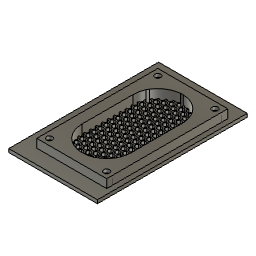
cover_side v6 (Autodesk Fusion 360 design; units mm, degrees)
Autodesk Fusion 360 part; units mm, degrees
(part 1 of 2)
sketch "Skizze1" plane through (0, 0, 0) normal (0, 0, 1) x (1, 0, 0)
  line L0 (26, -43.9) -> (-26, 43.9) construction
  line L1 (-26, -43.9) -> (26, 43.9) construction
  line L2 (21, -35.5) -> (-21, 35.5) construction
  line L3 (-21, -35.5) -> (21, 35.5) construction
  line L4 (23, -37.5) -> (-23, 37.5) construction
  line L5 (-23, -37.5) -> (23, 37.5) construction
  line L6 (0, 60) -> (0, -55) construction
  line L7 (16.75, -31.75) -> (-16.75, -31.75) construction
  line L8 (-16.75, -31.75) -> (-16.75, 31.75) construction
  line L9 (-16.75, 31.75) -> (16.75, 31.75) construction
  line L10 (16.75, 31.75) -> (16.75, -31.75) construction
  line L11 (16.75, -31.75) -> (-16.75, 31.75) construction
  line L12 (-16.75, -31.75) -> (16.75, 31.75) construction
  line L13 (20.5, -35.5) -> (-20.5, -35.5)
  line L14 (-20.5, -35.5) -> (-20.5, 35.5)
  line L15 (-20.5, 35.5) -> (20.5, 35.5)
  line L16 (20.5, 35.5) -> (20.5, -35.5)
  line L17 (20.5, -35.5) -> (-20.5, 35.5) construction
  line L18 (-20.5, -35.5) -> (20.5, 35.5) construction
  line L19 (-34.4017, -15) -> (37.5784, -15) construction
  line L20 (-32.2154, 15) -> (36.7375, 15) construction
  line L21 (14.5, -29.5) -> (-14.5, -29.5) construction
  line L22 (-14.5, -29.5) -> (-14.5, 29.5) construction
  line L23 (-14.5, 29.5) -> (14.5, 29.5) construction
  line L24 (14.5, 29.5) -> (14.5, -29.5) construction
  line L25 (14.5, -29.5) -> (-14.5, 29.5) construction
  line L26 (-14.5, -29.5) -> (14.5, 29.5) construction
  arc A0 (14.5, 15) -> (-14.5, 15) centre (0, 15) ccw
  arc A1 (-14.5, -15) -> (14.5, -15) centre (0, -15) ccw
  line L27 (-14.5, -15) -> (-14.5, 15)
  line L28 (14.5, -15) -> (14.5, 15)
  line L29 (-13.75, -30.799) -> (-13, -29.5)
  line L30 (-13, -29.5) -> (-13.75, -28.201)
  line L31 (-13.75, -28.201) -> (-15.25, -28.201)
  line L32 (-15.25, -28.201) -> (-16, -29.5)
  line L33 (-16, -29.5) -> (-15.25, -30.799)
  line L34 (-15.25, -30.799) -> (-13.75, -30.799)
  line L35 (-11.673, -26.8) -> (-11.673, -30.7) construction
  line L36 (-15, -27.75) -> (-9.3, -27.75) construction
  line L37 (-10.923, -29.049) -> (-10.173, -27.75)
  line L38 (-10.173, -27.75) -> (-10.923, -26.451)
  line L39 (-10.923, -26.451) -> (-12.423, -26.451)
  line L40 (-12.423, -26.451) -> (-13.173, -27.75)
  line L41 (-13.173, -27.75) -> (-12.423, -29.049)
  line L42 (-12.423, -29.049) -> (-10.923, -29.049)
  line L43 (-7.3455, -29.5) -> (-8.0955, -28.201)
  line L44 (-8.0955, -28.201) -> (-9.5955, -28.201)
  line L45 (-9.5955, -28.201) -> (-10.3455, -29.5)
  line L46 (-10.3455, -29.5) -> (-9.5955, -30.799)
  line L47 (-9.5955, -30.799) -> (-8.0955, -30.799)
  line L48 (-8.0955, -30.799) -> (-7.3455, -29.5)
  line L49 (-4.5185, -27.75) -> (-5.2685, -26.451)
  line L50 (-5.2685, -26.451) -> (-6.7685, -26.451)
  line L51 (-6.7685, -26.451) -> (-7.5185, -27.75)
  line L52 (-7.5185, -27.75) -> (-6.7685, -29.049)
  line L53 (-5.2685, -29.049) -> (-4.5185, -27.75)
  line L54 (-6.7685, -29.049) -> (-5.2685, -29.049)
  line L55 (-1.691, -29.5) -> (-2.441, -28.201)
  line L56 (-2.441, -28.201) -> (-3.941, -28.201)
  line L57 (-3.941, -28.201) -> (-4.691, -29.5)
  line L58 (-4.691, -29.5) -> (-3.941, -30.799)
  line L59 (-3.941, -30.799) -> (-2.441, -30.799)
  line L60 (-2.441, -30.799) -> (-1.691, -29.5)
  line L61 (1.136, -27.75) -> (0.386, -26.451)
  line L62 (0.386, -26.451) -> (-1.114, -26.451)
  line L63 (-1.114, -26.451) -> (-1.864, -27.75)
  line L64 (-1.864, -27.75) -> (-1.114, -29.049)
  line L65 (0.386, -29.049) -> (1.136, -27.75)
  line L66 (-1.114, -29.049) -> (0.386, -29.049)
  line L67 (3.9635, -29.5) -> (3.2135, -28.201)
  line L68 (3.2135, -28.201) -> (1.7135, -28.201)
  line L69 (1.7135, -28.201) -> (0.9635, -29.5)
  line L70 (0.9635, -29.5) -> (1.7135, -30.799)
  line L71 (1.7135, -30.799) -> (3.2135, -30.799)
  line L72 (3.2135, -30.799) -> (3.9635, -29.5)
  line L73 (6.7905, -27.75) -> (6.0405, -26.451)
  line L74 (6.0405, -26.451) -> (4.5405, -26.451)
  line L75 (4.5405, -26.451) -> (3.7905, -27.75)
  line L76 (3.7905, -27.75) -> (4.5405, -29.049)
  line L77 (6.0405, -29.049) -> (6.7905, -27.75)
  line L78 (4.5405, -29.049) -> (6.0405, -29.049)
  line L79 (9.618, -29.5) -> (8.868, -28.201)
  line L80 (8.868, -28.201) -> (7.368, -28.201)
  line L81 (7.368, -28.201) -> (6.618, -29.5)
  line L82 (6.618, -29.5) -> (7.368, -30.799)
  line L83 (7.368, -30.799) -> (8.868, -30.799)
  line L84 (8.868, -30.799) -> (9.618, -29.5)
  line L85 (12.445, -27.75) -> (11.695, -26.451)
  line L86 (11.695, -26.451) -> (10.195, -26.451)
  line L87 (10.195, -26.451) -> (9.445, -27.75)
  line L88 (9.445, -27.75) -> (10.195, -29.049)
  line L89 (11.695, -29.049) -> (12.445, -27.75)
  line L90 (10.195, -29.049) -> (11.695, -29.049)
  line L91 (15.2725, -29.5) -> (14.5225, -28.201)
  line L92 (14.5225, -28.201) -> (13.0225, -28.201)
  line L93 (13.0225, -28.201) -> (12.2725, -29.5)
  line L94 (12.2725, -29.5) -> (13.0225, -30.799)
  line L95 (13.0225, -30.799) -> (14.5225, -30.799)
  line L96 (14.5225, -30.799) -> (15.2725, -29.5)
  line L97 (18.0995, -27.75) -> (17.3495, -26.451)
  line L98 (17.3495, -26.451) -> (15.8495, -26.451)
  line L99 (15.8495, -26.451) -> (15.0995, -27.75)
  line L100 (15.0995, -27.75) -> (15.8495, -29.049)
  line L101 (17.3495, -29.049) -> (18.0995, -27.75)
  line L102 (15.8495, -29.049) -> (17.3495, -29.049)
  line L103 (-13, -26) -> (-13.75, -24.701)
  line L104 (-13.75, -24.701) -> (-15.25, -24.701)
  line L105 (-15.25, -24.701) -> (-16, -26)
  line L106 (-16, -26) -> (-15.25, -27.299)
  line L107 (-15.25, -27.299) -> (-13.75, -27.299)
  line L108 (-13.75, -27.299) -> (-13, -26)
  line L109 (-10.173, -24.25) -> (-10.923, -22.951)
  line L110 (-10.923, -22.951) -> (-12.423, -22.951)
  line L111 (-12.423, -22.951) -> (-13.173, -24.25)
  line L112 (-13.173, -24.25) -> (-12.423, -25.549)
  line L113 (-10.923, -25.549) -> (-10.173, -24.25)
  line L114 (-12.423, -25.549) -> (-10.923, -25.549)
  line L115 (-7.3455, -26) -> (-8.0955, -24.701)
  line L116 (-8.0955, -24.701) -> (-9.5955, -24.701)
  line L117 (-9.5955, -24.701) -> (-10.3455, -26)
  line L118 (-10.3455, -26) -> (-9.5955, -27.299)
  line L119 (-9.5955, -27.299) -> (-8.0955, -27.299)
  line L120 (-8.0955, -27.299) -> (-7.3455, -26)
  line L121 (-4.5185, -24.25) -> (-5.2685, -22.951)
  line L122 (-5.2685, -22.951) -> (-6.7685, -22.951)
  line L123 (-6.7685, -22.951) -> (-7.5185, -24.25)
  line L124 (-7.5185, -24.25) -> (-6.7685, -25.549)
  line L125 (-5.2685, -25.549) -> (-4.5185, -24.25)
  line L126 (-6.7685, -25.549) -> (-5.2685, -25.549)
  line L127 (-1.691, -26) -> (-2.441, -24.701)
  line L128 (-2.441, -24.701) -> (-3.941, -24.701)
  line L129 (-3.941, -24.701) -> (-4.691, -26)
  line L130 (-4.691, -26) -> (-3.941, -27.299)
  line L131 (-3.941, -27.299) -> (-2.441, -27.299)
  line L132 (-2.441, -27.299) -> (-1.691, -26)
  line L133 (1.136, -24.25) -> (0.386, -22.951)
  line L134 (0.386, -22.951) -> (-1.114, -22.951)
  line L135 (-1.114, -22.951) -> (-1.864, -24.25)
  line L136 (-1.864, -24.25) -> (-1.114, -25.549)
  line L137 (0.386, -25.549) -> (1.136, -24.25)
  line L138 (-1.114, -25.549) -> (0.386, -25.549)
  line L139 (3.9635, -26) -> (3.2135, -24.701)
  line L140 (3.2135, -24.701) -> (1.7135, -24.701)
  line L141 (1.7135, -24.701) -> (0.9635, -26)
  line L142 (0.9635, -26) -> (1.7135, -27.299)
  line L143 (1.7135, -27.299) -> (3.2135, -27.299)
  line L144 (3.2135, -27.299) -> (3.9635, -26)
  line L145 (6.7905, -24.25) -> (6.0405, -22.951)
  line L146 (6.0405, -22.951) -> (4.5405, -22.951)
  line L147 (4.5405, -22.951) -> (3.7905, -24.25)
  line L148 (3.7905, -24.25) -> (4.5405, -25.549)
  line L149 (6.0405, -25.549) -> (6.7905, -24.25)
  line L150 (4.5405, -25.549) -> (6.0405, -25.549)
  line L151 (9.618, -26) -> (8.868, -24.701)
  line L152 (8.868, -24.701) -> (7.368, -24.701)
  line L153 (7.368, -24.701) -> (6.618, -26)
  line L154 (6.618, -26) -> (7.368, -27.299)
  line L155 (7.368, -27.299) -> (8.868, -27.299)
  line L156 (8.868, -27.299) -> (9.618, -26)
  line L157 (12.445, -24.25) -> (11.695, -22.951)
  line L158 (11.695, -22.951) -> (10.195, -22.951)
  line L159 (10.195, -22.951) -> (9.445, -24.25)
  line L160 (9.445, -24.25) -> (10.195, -25.549)
  line L161 (11.695, -25.549) -> (12.445, -24.25)
  line L162 (10.195, -25.549) -> (11.695, -25.549)
  line L163 (15.2725, -26) -> (14.5225, -24.701)
  line L164 (14.5225, -24.701) -> (13.0225, -24.701)
  line L165 (13.0225, -24.701) -> (12.2725, -26)
  line L166 (12.2725, -26) -> (13.0225, -27.299)
  line L167 (13.0225, -27.299) -> (14.5225, -27.299)
  line L168 (14.5225, -27.299) -> (15.2725, -26)
  line L169 (18.0995, -24.25) -> (17.3495, -22.951)
  line L170 (17.3495, -22.951) -> (15.8495, -22.951)
  line L171 (15.8495, -22.951) -> (15.0995, -24.25)
  line L172 (15.0995, -24.25) -> (15.8495, -25.549)
  line L173 (17.3495, -25.549) -> (18.0995, -24.25)
  line L174 (15.8495, -25.549) -> (17.3495, -25.549)
  line L175 (-13, -22.5) -> (-13.75, -21.201)
  line L176 (-13.75, -21.201) -> (-15.25, -21.201)
  line L177 (-15.25, -21.201) -> (-16, -22.5)
  line L178 (-16, -22.5) -> (-15.25, -23.799)
  line L179 (-15.25, -23.799) -> (-13.75, -23.799)
  line L180 (-13.75, -23.799) -> (-13, -22.5)
  line L181 (-10.173, -20.75) -> (-10.923, -19.451)
  line L182 (-10.923, -19.451) -> (-12.423, -19.451)
  line L183 (-12.423, -19.451) -> (-13.173, -20.75)
  line L184 (-13.173, -20.75) -> (-12.423, -22.049)
  line L185 (-10.923, -22.049) -> (-10.173, -20.75)
  line L186 (-12.423, -22.049) -> (-10.923, -22.049)
  line L187 (-7.3455, -22.5) -> (-8.0955, -21.201)
  line L188 (-8.0955, -21.201) -> (-9.5955, -21.201)
  line L189 (-9.5955, -21.201) -> (-10.3455, -22.5)
  line L190 (-10.3455, -22.5) -> (-9.5955, -23.799)
  line L191 (-9.5955, -23.799) -> (-8.0955, -23.799)
  line L192 (-8.0955, -23.799) -> (-7.3455, -22.5)
  line L193 (-4.5185, -20.75) -> (-5.2685, -19.451)
  line L194 (-5.2685, -19.451) -> (-6.7685, -19.451)
  line L195 (-6.7685, -19.451) -> (-7.5185, -20.75)
  line L196 (-7.5185, -20.75) -> (-6.7685, -22.049)
  line L197 (-5.2685, -22.049) -> (-4.5185, -20.75)
  line L198 (-6.7685, -22.049) -> (-5.2685, -22.049)
  line L199 (-1.691, -22.5) -> (-2.441, -21.201)
  line L200 (-2.441, -21.201) -> (-3.941, -21.201)
  line L201 (-3.941, -21.201) -> (-4.691, -22.5)
  line L202 (-4.691, -22.5) -> (-3.941, -23.799)
  line L203 (-3.941, -23.799) -> (-2.441, -23.799)
  line L204 (-2.441, -23.799) -> (-1.691, -22.5)
  line L205 (1.136, -20.75) -> (0.386, -19.451)
  line L206 (0.386, -19.451) -> (-1.114, -19.451)
  line L207 (-1.114, -19.451) -> (-1.864, -20.75)
  line L208 (-1.864, -20.75) -> (-1.114, -22.049)
  line L209 (0.386, -22.049) -> (1.136, -20.75)
  line L210 (-1.114, -22.049) -> (0.386, -22.049)
  line L211 (3.9635, -22.5) -> (3.2135, -21.201)
  line L212 (3.2135, -21.201) -> (1.7135, -21.201)
  line L213 (1.7135, -21.201) -> (0.9635, -22.5)
  line L214 (0.9635, -22.5) -> (1.7135, -23.799)
  line L215 (1.7135, -23.799) -> (3.2135, -23.799)
  line L216 (3.2135, -23.799) -> (3.9635, -22.5)
  line L217 (6.7905, -20.75) -> (6.0405, -19.451)
  line L218 (6.0405, -19.451) -> (4.5405, -19.451)
  line L219 (4.5405, -19.451) -> (3.7905, -20.75)
  line L220 (3.7905, -20.75) -> (4.5405, -22.049)
  line L221 (6.0405, -22.049) -> (6.7905, -20.75)
  line L222 (4.5405, -22.049) -> (6.0405, -22.049)
  line L223 (9.618, -22.5) -> (8.868, -21.201)
  line L224 (8.868, -21.201) -> (7.368, -21.201)
  line L225 (7.368, -21.201) -> (6.618, -22.5)
  line L226 (6.618, -22.5) -> (7.368, -23.799)
  line L227 (7.368, -23.799) -> (8.868, -23.799)
  line L228 (8.868, -23.799) -> (9.618, -22.5)
  line L229 (12.445, -20.75) -> (11.695, -19.451)
  line L230 (11.695, -19.451) -> (10.195, -19.451)
  line L231 (10.195, -19.451) -> (9.445, -20.75)
  line L232 (9.445, -20.75) -> (10.195, -22.049)
  line L233 (11.695, -22.049) -> (12.445, -20.75)
  line L234 (10.195, -22.049) -> (11.695, -22.049)
  line L235 (15.2725, -22.5) -> (14.5225, -21.201)
  line L236 (14.5225, -21.201) -> (13.0225, -21.201)
  line L237 (13.0225, -21.201) -> (12.2725, -22.5)
  line L238 (12.2725, -22.5) -> (13.0225, -23.799)
  line L239 (13.0225, -23.799) -> (14.5225, -23.799)
  line L240 (14.5225, -23.799) -> (15.2725, -22.5)
  line L241 (18.0995, -20.75) -> (17.3495, -19.451)
  line L242 (17.3495, -19.451) -> (15.8495, -19.451)
  line L243 (15.8495, -19.451) -> (15.0995, -20.75)
  line L244 (15.0995, -20.75) -> (15.8495, -22.049)
  line L245 (17.3495, -22.049) -> (18.0995, -20.75)
  line L246 (15.8495, -22.049) -> (17.3495, -22.049)
  line L247 (-13, -19) -> (-13.75, -17.701)
  line L248 (-13.75, -17.701) -> (-15.25, -17.701)
  line L249 (-15.25, -17.701) -> (-16, -19)
  line L250 (-16, -19) -> (-15.25, -20.299)
  line L251 (-15.25, -20.299) -> (-13.75, -20.299)
  line L252 (-13.75, -20.299) -> (-13, -19)
  line L253 (-10.173, -17.25) -> (-10.923, -15.951)
  line L254 (-10.923, -15.951) -> (-12.423, -15.951)
  line L255 (-12.423, -15.951) -> (-13.173, -17.25)
  line L256 (-13.173, -17.25) -> (-12.423, -18.549)
  line L257 (-10.923, -18.549) -> (-10.173, -17.25)
  line L258 (-12.423, -18.549) -> (-10.923, -18.549)
  line L259 (-7.3455, -19) -> (-8.0955, -17.701)
  line L260 (-8.0955, -17.701) -> (-9.5955, -17.701)
  line L261 (-9.5955, -17.701) -> (-10.3455, -19)
  line L262 (-10.3455, -19) -> (-9.5955, -20.299)
  line L263 (-9.5955, -20.299) -> (-8.0955, -20.299)
  line L264 (-8.0955, -20.299) -> (-7.3455, -19)
  line L265 (-4.5185, -17.25) -> (-5.2685, -15.951)
  line L266 (-5.2685, -15.951) -> (-6.7685, -15.951)
  line L267 (-6.7685, -15.951) -> (-7.5185, -17.25)
  line L268 (-7.5185, -17.25) -> (-6.7685, -18.549)
  line L269 (-5.2685, -18.549) -> (-4.5185, -17.25)
  line L270 (-6.7685, -18.549) -> (-5.2685, -18.549)
  line L271 (-1.691, -19) -> (-2.441, -17.701)
  line L272 (-2.441, -17.701) -> (-3.941, -17.701)
  line L273 (-3.941, -17.701) -> (-4.691, -19)
  line L274 (-4.691, -19) -> (-3.941, -20.299)
  line L275 (-3.941, -20.299) -> (-2.441, -20.299)
  line L276 (-2.441, -20.299) -> (-1.691, -19)
  line L277 (1.136, -17.25) -> (0.386, -15.951)
  line L278 (0.386, -15.951) -> (-1.114, -15.951)
  line L279 (-1.114, -15.951) -> (-1.864, -17.25)
  line L280 (-1.864, -17.25) -> (-1.114, -18.549)
  line L281 (0.386, -18.549) -> (1.136, -17.25)
  line L282 (-1.114, -18.549) -> (0.386, -18.549)
  line L283 (3.9635, -19) -> (3.2135, -17.701)
  line L284 (3.2135, -17.701) -> (1.7135, -17.701)
  line L285 (1.7135, -17.701) -> (0.9635, -19)
  line L286 (0.9635, -19) -> (1.7135, -20.299)
  line L287 (1.7135, -20.299) -> (3.2135, -20.299)
  line L288 (3.2135, -20.299) -> (3.9635, -19)
  line L289 (6.7905, -17.25) -> (6.0405, -15.951)
  line L290 (6.0405, -15.951) -> (4.5405, -15.951)
  line L291 (4.5405, -15.951) -> (3.7905, -17.25)
  line L292 (3.7905, -17.25) -> (4.5405, -18.549)
  line L293 (6.0405, -18.549) -> (6.7905, -17.25)
  line L294 (4.5405, -18.549) -> (6.0405, -18.549)
  line L295 (9.618, -19) -> (8.868, -17.701)
  line L296 (8.868, -17.701) -> (7.368, -17.701)
  line L297 (7.368, -17.701) -> (6.618, -19)
  line L298 (6.618, -19) -> (7.368, -20.299)
  line L299 (7.368, -20.299) -> (8.868, -20.299)
  line L300 (8.868, -20.299) -> (9.618, -19)
  line L301 (12.445, -17.25) -> (11.695, -15.951)
  line L302 (11.695, -15.951) -> (10.195, -15.951)
  line L303 (10.195, -15.951) -> (9.445, -17.25)
  line L304 (9.445, -17.25) -> (10.195, -18.549)
  line L305 (11.695, -18.549) -> (12.445, -17.25)
  line L306 (10.195, -18.549) -> (11.695, -18.549)
  line L307 (15.2725, -19) -> (14.5225, -17.701)
  line L308 (14.5225, -17.701) -> (13.0225, -17.701)
  line L309 (13.0225, -17.701) -> (12.2725, -19)
  line L310 (12.2725, -19) -> (13.0225, -20.299)
  line L311 (13.0225, -20.299) -> (14.5225, -20.299)
  line L312 (14.5225, -20.299) -> (15.2725, -19)
  line L313 (18.0995, -17.25) -> (17.3495, -15.951)
  line L314 (17.3495, -15.951) -> (15.8495, -15.951)
  line L315 (15.8495, -15.951) -> (15.0995, -17.25)
  line L316 (15.0995, -17.25) -> (15.8495, -18.549)
  line L317 (17.3495, -18.549) -> (18.0995, -17.25)
  line L318 (15.8495, -18.549) -> (17.3495, -18.549)
  line L319 (-13, -15.5) -> (-13.75, -14.201)
  line L320 (-13.75, -14.201) -> (-15.25, -14.201)
  line L321 (-15.25, -14.201) -> (-16, -15.5)
  line L322 (-16, -15.5) -> (-15.25, -16.799)
  line L323 (-15.25, -16.799) -> (-13.75, -16.799)
  line L324 (-13.75, -16.799) -> (-13, -15.5)
  line L325 (-10.173, -13.75) -> (-10.923, -12.451)
  line L326 (-10.923, -12.451) -> (-12.423, -12.451)
  line L327 (-12.423, -12.451) -> (-13.173, -13.75)
  line L328 (-13.173, -13.75) -> (-12.423, -15.049)
  line L329 (-10.923, -15.049) -> (-10.173, -13.75)
  line L330 (-12.423, -15.049) -> (-10.923, -15.049)
  line L331 (-7.3455, -15.5) -> (-8.0955, -14.201)
  line L332 (-8.0955, -14.201) -> (-9.5955, -14.201)
  line L333 (-9.5955, -14.201) -> (-10.3455, -15.5)
  line L334 (-10.3455, -15.5) -> (-9.5955, -16.799)
  line L335 (-9.5955, -16.799) -> (-8.0955, -16.799)
  line L336 (-8.0955, -16.799) -> (-7.3455, -15.5)
  line L337 (-4.5185, -13.75) -> (-5.2685, -12.451)
  line L338 (-5.2685, -12.451) -> (-6.7685, -12.451)
  line L339 (-6.7685, -12.451) -> (-7.5185, -13.75)
  line L340 (-7.5185, -13.75) -> (-6.7685, -15.049)
  line L341 (-5.2685, -15.049) -> (-4.5185, -13.75)
  line L342 (-6.7685, -15.049) -> (-5.2685, -15.049)
  line L343 (-1.691, -15.5) -> (-2.441, -14.201)
  line L344 (-2.441, -14.201) -> (-3.941, -14.201)
  line L345 (-3.941, -14.201) -> (-4.691, -15.5)
  line L346 (-4.691, -15.5) -> (-3.941, -16.799)
  line L347 (-3.941, -16.799) -> (-2.441, -16.799)
  line L348 (-2.441, -16.799) -> (-1.691, -15.5)
  line L349 (1.136, -13.75) -> (0.386, -12.451)
  line L350 (0.386, -12.451) -> (-1.114, -12.451)
  line L351 (-1.114, -12.451) -> (-1.864, -13.75)
  line L352 (-1.864, -13.75) -> (-1.114, -15.049)
  line L353 (0.386, -15.049) -> (1.136, -13.75)
  line L354 (-1.114, -15.049) -> (0.386, -15.049)
  line L355 (3.9635, -15.5) -> (3.2135, -14.201)
  line L356 (3.2135, -14.201) -> (1.7135, -14.201)
  line L357 (1.7135, -14.201) -> (0.9635, -15.5)
  line L358 (0.9635, -15.5) -> (1.7135, -16.799)
  line L359 (1.7135, -16.799) -> (3.2135, -16.799)
  line L360 (3.2135, -16.799) -> (3.9635, -15.5)
  line L361 (6.7905, -13.75) -> (6.0405, -12.451)
  line L362 (6.0405, -12.451) -> (4.5405, -12.451)
  line L363 (4.5405, -12.451) -> (3.7905, -13.75)
  line L364 (3.7905, -13.75) -> (4.5405, -15.049)
  line L365 (6.0405, -15.049) -> (6.7905, -13.75)
  line L366 (4.5405, -15.049) -> (6.0405, -15.049)
  line L367 (9.618, -15.5) -> (8.868, -14.201)
  line L368 (8.868, -14.201) -> (7.368, -14.201)
  line L369 (7.368, -14.201) -> (6.618, -15.5)
  line L370 (6.618, -15.5) -> (7.368, -16.799)
  line L371 (7.368, -16.799) -> (8.868, -16.799)
  line L372 (8.868, -16.799) -> (9.618, -15.5)
  line L373 (12.445, -13.75) -> (11.695, -12.451)
  line L374 (11.695, -12.451) -> (10.195, -12.451)
  line L375 (10.195, -12.451) -> (9.445, -13.75)
  line L376 (9.445, -13.75) -> (10.195, -15.049)
  line L377 (11.695, -15.049) -> (12.445, -13.75)
  line L378 (10.195, -15.049) -> (11.695, -15.049)
  line L379 (15.2725, -15.5) -> (14.5225, -14.201)
  line L380 (14.5225, -14.201) -> (13.0225, -14.201)
  line L381 (13.0225, -14.201) -> (12.2725, -15.5)
  line L382 (12.2725, -15.5) -> (13.0225, -16.799)
  line L383 (13.0225, -16.799) -> (14.5225, -16.799)
  line L384 (14.5225, -16.799) -> (15.2725, -15.5)
  line L385 (18.0995, -13.75) -> (17.3495, -12.451)
  line L386 (17.3495, -12.451) -> (15.8495, -12.451)
  line L387 (15.8495, -12.451) -> (15.0995, -13.75)
  line L388 (15.0995, -13.75) -> (15.8495, -15.049)
  line L389 (17.3495, -15.049) -> (18.0995, -13.75)
  line L390 (15.8495, -15.049) -> (17.3495, -15.049)
  line L391 (-13, -12) -> (-13.75, -10.701)
  line L392 (-13.75, -10.701) -> (-15.25, -10.701)
  line L393 (-15.25, -10.701) -> (-16, -12)
  line L394 (-16, -12) -> (-15.25, -13.299)
  line L395 (-15.25, -13.299) -> (-13.75, -13.299)
  line L396 (-13.75, -13.299) -> (-13, -12)
  line L397 (-10.173, -10.25) -> (-10.923, -8.951)
  line L398 (-10.923, -8.951) -> (-12.423, -8.951)
  line L399 (-12.423, -8.951) -> (-13.173, -10.25)
  line L400 (-13.173, -10.25) -> (-12.423, -11.549)
  line L401 (-10.923, -11.549) -> (-10.173, -10.25)
  line L402 (-12.423, -11.549) -> (-10.923, -11.549)
  line L403 (-7.3455, -12) -> (-8.0955, -10.701)
  line L404 (-8.0955, -10.701) -> (-9.5955, -10.701)
  line L405 (-9.5955, -10.701) -> (-10.3455, -12)
  line L406 (-10.3455, -12) -> (-9.5955, -13.299)
  line L407 (-9.5955, -13.299) -> (-8.0955, -13.299)
  line L408 (-8.0955, -13.299) -> (-7.3455, -12)
  line L409 (-4.5185, -10.25) -> (-5.2685, -8.951)
  line L410 (-5.2685, -8.951) -> (-6.7685, -8.951)
  line L411 (-6.7685, -8.951) -> (-7.5185, -10.25)
  line L412 (-7.5185, -10.25) -> (-6.7685, -11.549)
  line L413 (-5.2685, -11.549) -> (-4.5185, -10.25)
  line L414 (-6.7685, -11.549) -> (-5.2685, -11.549)
  line L415 (-1.691, -12) -> (-2.441, -10.701)
  line L416 (-2.441, -10.701) -> (-3.941, -10.701)
  line L417 (-3.941, -10.701) -> (-4.691, -12)
  line L418 (-4.691, -12) -> (-3.941, -13.299)
  line L419 (-3.941, -13.299) -> (-2.441, -13.299)
  line L420 (-2.441, -13.299) -> (-1.691, -12)
  line L421 (1.136, -10.25) -> (0.386, -8.951)
  line L422 (0.386, -8.951) -> (-1.114, -8.951)
  line L423 (-1.114, -8.951) -> (-1.864, -10.25)
  line L424 (-1.864, -10.25) -> (-1.114, -11.549)
  line L425 (0.386, -11.549) -> (1.136, -10.25)
  line L426 (-1.114, -11.549) -> (0.386, -11.549)
  line L427 (3.9635, -12) -> (3.2135, -10.701)
  line L428 (3.2135, -10.701) -> (1.7135, -10.701)
  line L429 (1.7135, -10.701) -> (0.9635, -12)
  line L430 (0.9635, -12) -> (1.7135, -13.299)
  line L431 (1.7135, -13.299) -> (3.2135, -13.299)
  line L432 (3.2135, -13.299) -> (3.9635, -12)
  line L433 (6.7905, -10.25) -> (6.0405, -8.951)
  line L434 (6.0405, -8.951) -> (4.5405, -8.951)
  line L435 (4.5405, -8.951) -> (3.7905, -10.25)
  line L436 (3.7905, -10.25) -> (4.5405, -11.549)
  line L437 (6.0405, -11.549) -> (6.7905, -10.25)
  line L438 (4.5405, -11.549) -> (6.0405, -11.549)
  line L439 (9.618, -12) -> (8.868, -10.701)
  line L440 (8.868, -10.701) -> (7.368, -10.701)
  line L441 (7.368, -10.701) -> (6.618, -12)
  line L442 (6.618, -12) -> (7.368, -13.299)
  line L443 (7.368, -13.299) -> (8.868, -13.299)
  line L444 (8.868, -13.299) -> (9.618, -12)
  line L445 (12.445, -10.25) -> (11.695, -8.951)
  line L446 (11.695, -8.951) -> (10.195, -8.951)
  line L447 (10.195, -8.951) -> (9.445, -10.25)
  line L448 (9.445, -10.25) -> (10.195, -11.549)
  line L449 (11.695, -11.549) -> (12.445, -10.25)
  line L450 (10.195, -11.549) -> (11.695, -11.549)
  line L451 (15.2725, -12) -> (14.5225, -10.701)
  line L452 (14.5225, -10.701) -> (13.0225, -10.701)
  line L453 (13.0225, -10.701) -> (12.2725, -12)
  line L454 (12.2725, -12) -> (13.0225, -13.299)
  line L455 (13.0225, -13.299) -> (14.5225, -13.299)
  line L456 (14.5225, -13.299) -> (15.2725, -12)
  line L457 (18.0995, -10.25) -> (17.3495, -8.951)
  line L458 (17.3495, -8.951) -> (15.8495, -8.951)
  line L459 (15.8495, -8.951) -> (15.0995, -10.25)
  line L460 (15.0995, -10.25) -> (15.8495, -11.549)
  line L461 (17.3495, -11.549) -> (18.0995, -10.25)
  line L462 (15.8495, -11.549) -> (17.3495, -11.549)
  line L463 (-13, -8.5) -> (-13.75, -7.201)
  line L464 (-13.75, -7.201) -> (-15.25, -7.201)
  line L465 (-15.25, -7.201) -> (-16, -8.5)
  line L466 (-16, -8.5) -> (-15.25, -9.799)
  line L467 (-15.25, -9.799) -> (-13.75, -9.799)
  line L468 (-13.75, -9.799) -> (-13, -8.5)
  line L469 (-10.173, -6.75) -> (-10.923, -5.451)
  line L470 (-10.923, -5.451) -> (-12.423, -5.451)
  line L471 (-12.423, -5.451) -> (-13.173, -6.75)
  line L472 (-13.173, -6.75) -> (-12.423, -8.049)
  line L473 (-10.923, -8.049) -> (-10.173, -6.75)
  line L474 (-12.423, -8.049) -> (-10.923, -8.049)
  line L475 (-7.3455, -8.5) -> (-8.0955, -7.201)
  line L476 (-8.0955, -7.201) -> (-9.5955, -7.201)
  line L477 (-9.5955, -7.201) -> (-10.3455, -8.5)
  line L478 (-10.3455, -8.5) -> (-9.5955, -9.799)
  line L479 (-9.5955, -9.799) -> (-8.0955, -9.799)
  line L480 (-8.0955, -9.799) -> (-7.3455, -8.5)
  line L481 (-4.5185, -6.75) -> (-5.2685, -5.451)
  line L482 (-5.2685, -5.451) -> (-6.7685, -5.451)
  line L483 (-6.7685, -5.451) -> (-7.5185, -6.75)
  line L484 (-7.5185, -6.75) -> (-6.7685, -8.049)
  line L485 (-5.2685, -8.049) -> (-4.5185, -6.75)
  line L486 (-6.7685, -8.049) -> (-5.2685, -8.049)
  line L487 (-1.691, -8.5) -> (-2.441, -7.201)
  line L488 (-2.441, -7.201) -> (-3.941, -7.201)
  line L489 (-3.941, -7.201) -> (-4.691, -8.5)
  line L490 (-4.691, -8.5) -> (-3.941, -9.799)
  line L491 (-3.941, -9.799) -> (-2.441, -9.799)
  line L492 (-2.441, -9.799) -> (-1.691, -8.5)
  line L493 (1.136, -6.75) -> (0.386, -5.451)
  line L494 (0.386, -5.451) -> (-1.114, -5.451)
  line L495 (-1.114, -5.451) -> (-1.864, -6.75)
  line L496 (-1.864, -6.75) -> (-1.114, -8.049)
  line L497 (0.386, -8.049) -> (1.136, -6.75)
  line L498 (-1.114, -8.049) -> (0.386, -8.049)
  line L499 (3.9635, -8.5) -> (3.2135, -7.201)
  line L500 (3.2135, -7.201) -> (1.7135, -7.201)
  line L501 (1.7135, -7.201) -> (0.9635, -8.5)
  line L502 (0.9635, -8.5) -> (1.7135, -9.799)
  line L503 (1.7135, -9.799) -> (3.2135, -9.799)
  line L504 (3.2135, -9.799) -> (3.9635, -8.5)
  line L505 (6.7905, -6.75) -> (6.0405, -5.451)
  line L506 (6.0405, -5.451) -> (4.5405, -5.451)
  line L507 (4.5405, -5.451) -> (3.7905, -6.75)
  line L508 (3.7905, -6.75) -> (4.5405, -8.049)
  line L509 (6.0405, -8.049) -> (6.7905, -6.75)
  line L510 (4.5405, -8.049) -> (6.0405, -8.049)
  line L511 (9.618, -8.5) -> (8.868, -7.201)
  line L512 (8.868, -7.201) -> (7.368, -7.201)
  line L513 (7.368, -7.201) -> (6.618, -8.5)
  line L514 (6.618, -8.5) -> (7.368, -9.799)
  line L515 (7.368, -9.799) -> (8.868, -9.799)
  line L516 (8.868, -9.799) -> (9.618, -8.5)
  line L517 (12.445, -6.75) -> (11.695, -5.451)
  line L518 (11.695, -5.451) -> (10.195, -5.451)
  line L519 (10.195, -5.451) -> (9.445, -6.75)
  line L520 (9.445, -6.75) -> (10.195, -8.049)
  line L521 (11.695, -8.049) -> (12.445, -6.75)
  line L522 (10.195, -8.049) -> (11.695, -8.049)
  line L523 (15.2725, -8.5) -> (14.5225, -7.201)
  line L524 (14.5225, -7.201) -> (13.0225, -7.201)
  line L525 (13.0225, -7.201) -> (12.2725, -8.5)
  line L526 (12.2725, -8.5) -> (13.0225, -9.799)
  line L527 (13.0225, -9.799) -> (14.5225, -9.799)
  line L528 (14.5225, -9.799) -> (15.2725, -8.5)
  line L529 (18.0995, -6.75) -> (17.3495, -5.451)
  line L530 (17.3495, -5.451) -> (15.8495, -5.451)
  line L531 (15.8495, -5.451) -> (15.0995, -6.75)
  line L532 (15.0995, -6.75) -> (15.8495, -8.049)
  line L533 (17.3495, -8.049) -> (18.0995, -6.75)
  line L534 (15.8495, -8.049) -> (17.3495, -8.049)
  line L535 (-13, -5) -> (-13.75, -3.701)
  line L536 (-13.75, -3.701) -> (-15.25, -3.701)
  line L537 (-15.25, -3.701) -> (-16, -5)
  line L538 (-16, -5) -> (-15.25, -6.299)
  line L539 (-15.25, -6.299) -> (-13.75, -6.299)
  line L540 (-13.75, -6.299) -> (-13, -5)
  line L541 (-10.173, -3.25) -> (-10.923, -1.951)
  line L542 (-10.923, -1.951) -> (-12.423, -1.951)
  line L543 (-12.423, -1.951) -> (-13.173, -3.25)
  line L544 (-13.173, -3.25) -> (-12.423, -4.549)
  line L545 (-10.923, -4.549) -> (-10.173, -3.25)
  line L546 (-12.423, -4.549) -> (-10.923, -4.549)
  line L547 (-7.3455, -5) -> (-8.0955, -3.701)
  line L548 (-8.0955, -3.701) -> (-9.5955, -3.701)
  line L549 (-9.5955, -3.701) -> (-10.3455, -5)
  line L550 (-10.3455, -5) -> (-9.5955, -6.299)
  line L551 (-9.5955, -6.299) -> (-8.0955, -6.299)
  line L552 (-8.0955, -6.299) -> (-7.3455, -5)
  line L553 (-4.5185, -3.25) -> (-5.2685, -1.951)
  line L554 (-5.2685, -1.951) -> (-6.7685, -1.951)
  line L555 (-6.7685, -1.951) -> (-7.5185, -3.25)
  line L556 (-7.5185, -3.25) -> (-6.7685, -4.549)
  line L557 (-5.2685, -4.549) -> (-4.5185, -3.25)
  line L558 (-6.7685, -4.549) -> (-5.2685, -4.549)
  line L559 (-1.691, -5) -> (-2.441, -3.701)
  line L560 (-2.441, -3.701) -> (-3.941, -3.701)
  line L561 (-3.941, -3.701) -> (-4.691, -5)
  line L562 (-4.691, -5) -> (-3.941, -6.299)
  line L563 (-3.941, -6.299) -> (-2.441, -6.299)
  line L564 (-2.441, -6.299) -> (-1.691, -5)
  line L565 (1.136, -3.25) -> (0.386, -1.951)
  line L566 (0.386, -1.951) -> (-1.114, -1.951)
  line L567 (-1.114, -1.951) -> (-1.864, -3.25)
  line L568 (-1.864, -3.25) -> (-1.114, -4.549)
  line L569 (0.386, -4.549) -> (1.136, -3.25)
  line L570 (-1.114, -4.549) -> (0.386, -4.549)
  line L571 (3.9635, -5) -> (3.2135, -3.701)
  line L572 (3.2135, -3.701) -> (1.7135, -3.701)
  line L573 (1.7135, -3.701) -> (0.9635, -5)
  line L574 (0.9635, -5) -> (1.7135, -6.299)
  line L575 (1.7135, -6.299) -> (3.2135, -6.299)
  line L576 (3.2135, -6.299) -> (3.9635, -5)
  line L577 (6.7905, -3.25) -> (6.0405, -1.951)
  line L578 (6.0405, -1.951) -> (4.5405, -1.951)
  line L579 (4.5405, -1.951) -> (3.7905, -3.25)
  line L580 (3.7905, -3.25) -> (4.5405, -4.549)
  line L581 (6.0405, -4.549) -> (6.7905, -3.25)
  line L582 (4.5405, -4.549) -> (6.0405, -4.549)
  line L583 (9.618, -5) -> (8.868, -3.701)
  line L584 (8.868, -3.701) -> (7.368, -3.701)
  line L585 (7.368, -3.701) -> (6.618, -5)
  line L586 (6.618, -5) -> (7.368, -6.299)
  line L587 (7.368, -6.299) -> (8.868, -6.299)
  line L588 (8.868, -6.299) -> (9.618, -5)
  line L589 (12.445, -3.25) -> (11.695, -1.951)
  line L590 (11.695, -1.951) -> (10.195, -1.951)
  line L591 (10.195, -1.951) -> (9.445, -3.25)
  line L592 (9.445, -3.25) -> (10.195, -4.549)
  line L593 (11.695, -4.549) -> (12.445, -3.25)
  line L594 (10.195, -4.549) -> (11.695, -4.549)
  line L595 (15.2725, -5) -> (14.5225, -3.701)
  line L596 (14.5225, -3.701) -> (13.0225, -3.701)
  line L597 (13.0225, -3.701) -> (12.2725, -5)
  line L598 (12.2725, -5) -> (13.0225, -6.299)
  line L599 (13.0225, -6.299) -> (14.5225, -6.299)
  line L600 (14.5225, -6.299) -> (15.2725, -5)
  line L601 (18.0995, -3.25) -> (17.3495, -1.951)
  line L602 (17.3495, -1.951) -> (15.8495, -1.951)
  line L603 (15.8495, -1.951) -> (15.0995, -3.25)
  line L604 (15.0995, -3.25) -> (15.8495, -4.549)
  line L605 (17.3495, -4.549) -> (18.0995, -3.25)
  line L606 (15.8495, -4.549) -> (17.3495, -4.549)
  line L607 (-13, -1.5) -> (-13.75, -0.201)
  line L608 (-13.75, -0.201) -> (-15.25, -0.201)
  line L609 (-15.25, -0.201) -> (-16, -1.5)
  line L610 (-16, -1.5) -> (-15.25, -2.799)
  line L611 (-15.25, -2.799) -> (-13.75, -2.799)
  line L612 (-13.75, -2.799) -> (-13, -1.5)
  line L613 (-10.173, 0.25) -> (-10.923, 1.549)
  line L614 (-10.923, 1.549) -> (-12.423, 1.549)
  line L615 (-12.423, 1.549) -> (-13.173, 0.25)
  line L616 (-13.173, 0.25) -> (-12.423, -1.049)
  line L617 (-10.923, -1.049) -> (-10.173, 0.25)
  line L618 (-12.423, -1.049) -> (-10.923, -1.049)
  line L619 (-7.3455, -1.5) -> (-8.0955, -0.201)
  line L620 (-8.0955, -0.201) -> (-9.5955, -0.201)
  line L621 (-9.5955, -0.201) -> (-10.3455, -1.5)
  line L622 (-10.3455, -1.5) -> (-9.5955, -2.799)
  line L623 (-9.5955, -2.799) -> (-8.0955, -2.799)
  line L624 (-8.0955, -2.799) -> (-7.3455, -1.5)
  line L625 (-4.5185, 0.25) -> (-5.2685, 1.549)
  line L626 (-5.2685, 1.549) -> (-6.7685, 1.549)
  line L627 (-6.7685, 1.549) -> (-7.5185, 0.25)
  line L628 (-7.5185, 0.25) -> (-6.7685, -1.049)
  line L629 (-5.2685, -1.049) -> (-4.5185, 0.25)
  line L630 (-6.7685, -1.049) -> (-5.2685, -1.049)
  line L631 (-1.691, -1.5) -> (-2.441, -0.201)
  line L632 (-2.441, -0.201) -> (-3.941, -0.201)
  line L633 (-3.941, -0.201) -> (-4.691, -1.5)
  line L634 (-4.691, -1.5) -> (-3.941, -2.799)
  line L635 (-3.941, -2.799) -> (-2.441, -2.799)
  line L636 (-2.441, -2.799) -> (-1.691, -1.5)
  line L637 (1.136, 0.25) -> (0.386, 1.549)
  line L638 (0.386, 1.549) -> (-1.114, 1.549)
  line L639 (-1.114, 1.549) -> (-1.864, 0.25)
  line L640 (-1.864, 0.25) -> (-1.114, -1.049)
  line L641 (0.386, -1.049) -> (1.136, 0.25)
  line L642 (-1.114, -1.049) -> (0.386, -1.049)
  line L643 (3.9635, -1.5) -> (3.2135, -0.201)
  line L644 (3.2135, -0.201) -> (1.7135, -0.201)
  line L645 (1.7135, -0.201) -> (0.9635, -1.5)
  line L646 (0.9635, -1.5) -> (1.7135, -2.799)
  line L647 (1.7135, -2.799) -> (3.2135, -2.799)
  line L648 (3.2135, -2.799) -> (3.9635, -1.5)
  line L649 (6.7905, 0.25) -> (6.0405, 1.549)
  line L650 (6.0405, 1.549) -> (4.5405, 1.549)
  line L651 (4.5405, 1.549) -> (3.7905, 0.25)
  line L652 (3.7905, 0.25) -> (4.5405, -1.049)
  line L653 (6.0405, -1.049) -> (6.7905, 0.25)
  line L654 (4.5405, -1.049) -> (6.0405, -1.049)
  line L655 (9.618, -1.5) -> (8.868, -0.201)
  line L656 (8.868, -0.201) -> (7.368, -0.201)
  line L657 (7.368, -0.201) -> (6.618, -1.5)
  line L658 (6.618, -1.5) -> (7.368, -2.799)
  line L659 (7.368, -2.799) -> (8.868, -2.799)
  line L660 (8.868, -2.799) -> (9.618, -1.5)
  line L661 (12.445, 0.25) -> (11.695, 1.549)
  line L662 (11.695, 1.549) -> (10.195, 1.549)
  line L663 (10.195, 1.549) -> (9.445, 0.25)
  line L664 (9.445, 0.25) -> (10.195, -1.049)
  line L665 (11.695, -1.049) -> (12.445, 0.25)
  line L666 (10.195, -1.049) -> (11.695, -1.049)
  line L667 (15.2725, -1.5) -> (14.5225, -0.201)
  line L668 (14.5225, -0.201) -> (13.0225, -0.201)
  line L669 (13.0225, -0.201) -> (12.2725, -1.5)
  line L670 (12.2725, -1.5) -> (13.0225, -2.799)
  line L671 (13.0225, -2.799) -> (14.5225, -2.799)
  line L672 (14.5225, -2.799) -> (15.2725, -1.5)
  line L673 (18.0995, 0.25) -> (17.3495, 1.549)
  line L674 (17.3495, 1.549) -> (15.8495, 1.549)
  line L675 (15.8495, 1.549) -> (15.0995, 0.25)
  line L676 (15.0995, 0.25) -> (15.8495, -1.049)
  line L677 (17.3495, -1.049) -> (18.0995, 0.25)
  line L678 (15.8495, -1.049) -> (17.3495, -1.049)
  line L679 (-13, 2) -> (-13.75, 3.299)
  line L680 (-13.75, 3.299) -> (-15.25, 3.299)
  line L681 (-15.25, 3.299) -> (-16, 2)
  line L682 (-16, 2) -> (-15.25, 0.701)
  line L683 (-15.25, 0.701) -> (-13.75, 0.701)
  line L684 (-13.75, 0.701) -> (-13, 2)
  line L685 (-10.173, 3.75) -> (-10.923, 5.049)
  line L686 (-10.923, 5.049) -> (-12.423, 5.049)
  line L687 (-12.423, 5.049) -> (-13.173, 3.75)
  line L688 (-13.173, 3.75) -> (-12.423, 2.451)
  line L689 (-10.923, 2.451) -> (-10.173, 3.75)
  line L690 (-12.423, 2.451) -> (-10.923, 2.451)
  line L691 (-7.3455, 2) -> (-8.0955, 3.299)
  line L692 (-8.0955, 3.299) -> (-9.5955, 3.299)
  line L693 (-9.5955, 3.299) -> (-10.3455, 2)
  line L694 (-10.3455, 2) -> (-9.5955, 0.701)
  line L695 (-9.5955, 0.701) -> (-8.0955, 0.701)
  line L696 (-8.0955, 0.701) -> (-7.3455, 2)
  line L697 (-4.5185, 3.75) -> (-5.2685, 5.049)
  line L698 (-5.2685, 5.049) -> (-6.7685, 5.049)
  line L699 (-6.7685, 5.049) -> (-7.5185, 3.75)
  line L700 (-7.5185, 3.75) -> (-6.7685, 2.451)
  line L701 (-5.2685, 2.451) -> (-4.5185, 3.75)
  line L702 (-6.7685, 2.451) -> (-5.2685, 2.451)
  line L703 (-1.691, 2) -> (-2.441, 3.299)
  line L704 (-2.441, 3.299) -> (-3.941, 3.299)
  line L705 (-3.941, 3.299) -> (-4.691, 2)
  line L706 (-4.691, 2) -> (-3.941, 0.701)
  line L707 (-3.941, 0.701) -> (-2.441, 0.701)
  line L708 (-2.441, 0.701) -> (-1.691, 2)
  line L709 (1.136, 3.75) -> (0.386, 5.049)
  line L710 (0.386, 5.049) -> (-1.114, 5.049)
  line L711 (-1.114, 5.049) -> (-1.864, 3.75)
  line L712 (-1.864, 3.75) -> (-1.114, 2.451)
  line L713 (0.386, 2.451) -> (1.136, 3.75)
  line L714 (-1.114, 2.451) -> (0.386, 2.451)
  line L715 (3.9635, 2) -> (3.2135, 3.299)
  line L716 (3.2135, 3.299) -> (1.7135, 3.299)
  line L717 (1.7135, 3.299) -> (0.9635, 2)
  line L718 (0.9635, 2) -> (1.7135, 0.701)
  line L719 (1.7135, 0.701) -> (3.2135, 0.701)
  line L720 (3.2135, 0.701) -> (3.9635, 2)
  line L721 (6.7905, 3.75) -> (6.0405, 5.049)
  line L722 (6.0405, 5.049) -> (4.5405, 5.049)
  line L723 (4.5405, 5.049) -> (3.7905, 3.75)
  line L724 (3.7905, 3.75) -> (4.5405, 2.451)
  line L725 (6.0405, 2.451) -> (6.7905, 3.75)
  line L726 (4.5405, 2.451) -> (6.0405, 2.451)
  line L727 (9.618, 2) -> (8.868, 3.299)
  line L728 (8.868, 3.299) -> (7.368, 3.299)
  line L729 (7.368, 3.299) -> (6.618, 2)
  line L730 (6.618, 2) -> (7.368, 0.701)
  line L731 (7.368, 0.701) -> (8.868, 0.701)
  line L732 (8.868, 0.701) -> (9.618, 2)
  line L733 (12.445, 3.75) -> (11.695, 5.049)
  line L734 (11.695, 5.049) -> (10.195, 5.049)
  line L735 (10.195, 5.049) -> (9.445, 3.75)
  line L736 (9.445, 3.75) -> (10.195, 2.451)
  line L737 (11.695, 2.451) -> (12.445, 3.75)
  line L738 (10.195, 2.451) -> (11.695, 2.451)
  line L739 (15.2725, 2) -> (14.5225, 3.299)
  line L740 (14.5225, 3.299) -> (13.0225, 3.299)
  line L741 (13.0225, 3.299) -> (12.2725, 2)
  line L742 (12.2725, 2) -> (13.0225, 0.701)
  line L743 (13.0225, 0.701) -> (14.5225, 0.701)
  line L744 (14.5225, 0.701) -> (15.2725, 2)
  line L745 (18.0995, 3.75) -> (17.3495, 5.049)
  line L746 (17.3495, 5.049) -> (15.8495, 5.049)
  line L747 (15.8495, 5.049) -> (15.0995, 3.75)
  line L748 (15.0995, 3.75) -> (15.8495, 2.451)
  line L749 (17.3495, 2.451) -> (18.0995, 3.75)
  line L750 (15.8495, 2.451) -> (17.3495, 2.451)
  line L751 (-13, 5.5) -> (-13.75, 6.799)
  line L752 (-13.75, 6.799) -> (-15.25, 6.799)
  line L753 (-15.25, 6.799) -> (-16, 5.5)
  line L754 (-16, 5.5) -> (-15.25, 4.201)
  line L755 (-15.25, 4.201) -> (-13.75, 4.201)
  line L756 (-13.75, 4.201) -> (-13, 5.5)
  line L757 (-10.173, 7.25) -> (-10.923, 8.549)
  line L758 (-10.923, 8.549) -> (-12.423, 8.549)
  line L759 (-12.423, 8.549) -> (-13.173, 7.25)
  line L760 (-13.173, 7.25) -> (-12.423, 5.951)
  line L761 (-10.923, 5.951) -> (-10.173, 7.25)
  line L762 (-12.423, 5.951) -> (-10.923, 5.951)
  line L763 (-7.3455, 5.5) -> (-8.0955, 6.799)
  line L764 (-8.0955, 6.799) -> (-9.5955, 6.799)
  line L765 (-9.5955, 6.799) -> (-10.3455, 5.5)
  line L766 (-10.3455, 5.5) -> (-9.5955, 4.201)
  line L767 (-9.5955, 4.201) -> (-8.0955, 4.201)
  line L768 (-8.0955, 4.201) -> (-7.3455, 5.5)
  line L769 (-4.5185, 7.25) -> (-5.2685, 8.549)
  line L770 (-5.2685, 8.549) -> (-6.7685, 8.549)
  line L771 (-6.7685, 8.549) -> (-7.5185, 7.25)
  line L772 (-7.5185, 7.25) -> (-6.7685, 5.951)
  line L773 (-5.2685, 5.951) -> (-4.5185, 7.25)
  line L774 (-6.7685, 5.951) -> (-5.2685, 5.951)
  line L775 (-1.691, 5.5) -> (-2.441, 6.799)
  line L776 (-2.441, 6.799) -> (-3.941, 6.799)
  line L777 (-3.941, 6.799) -> (-4.691, 5.5)
  line L778 (-4.691, 5.5) -> (-3.941, 4.201)
  line L779 (-3.941, 4.201) -> (-2.441, 4.201)
  line L780 (-2.441, 4.201) -> (-1.691, 5.5)
  line L781 (1.136, 7.25) -> (0.386, 8.549)
  line L782 (0.386, 8.549) -> (-1.114, 8.549)
  line L783 (-1.114, 8.549) -> (-1.864, 7.25)
  line L784 (-1.864, 7.25) -> (-1.114, 5.951)
  line L785 (0.386, 5.951) -> (1.136, 7.25)
  line L786 (-1.114, 5.951) -> (0.386, 5.951)
  line L787 (3.9635, 5.5) -> (3.2135, 6.799)
  line L788 (3.2135, 6.799) -> (1.7135, 6.799)
  line L789 (1.7135, 6.799) -> (0.9635, 5.5)
  line L790 (0.9635, 5.5) -> (1.7135, 4.201)
  line L791 (1.7135, 4.201) -> (3.2135, 4.201)
  line L792 (3.2135, 4.201) -> (3.9635, 5.5)
  line L793 (6.7905, 7.25) -> (6.0405, 8.549)
  line L794 (6.0405, 8.549) -> (4.5405, 8.549)
  line L795 (4.5405, 8.549) -> (3.7905, 7.25)
  line L796 (3.7905, 7.25) -> (4.5405, 5.951)
  line L797 (6.0405, 5.951) -> (6.7905, 7.25)
  line L798 (4.5405, 5.951) -> (6.0405, 5.951)
  line L799 (9.618, 5.5) -> (8.868, 6.799)
  line L800 (8.868, 6.799) -> (7.368, 6.799)
  line L801 (7.368, 6.799) -> (6.618, 5.5)
  line L802 (6.618, 5.5) -> (7.368, 4.201)
  line L803 (7.368, 4.201) -> (8.868, 4.201)
  line L804 (8.868, 4.201) -> (9.618, 5.5)
  line L805 (12.445, 7.25) -> (11.695, 8.549)
  line L806 (11.695, 8.549) -> (10.195, 8.549)
  line L807 (10.195, 8.549) -> (9.445, 7.25)
  line L808 (9.445, 7.25) -> (10.195, 5.951)
  line L809 (11.695, 5.951) -> (12.445, 7.25)
  line L810 (10.195, 5.951) -> (11.695, 5.951)
  line L811 (15.2725, 5.5) -> (14.5225, 6.799)
  line L812 (14.5225, 6.799) -> (13.0225, 6.799)
  line L813 (13.0225, 6.799) -> (12.2725, 5.5)
  line L814 (12.2725, 5.5) -> (13.0225, 4.201)
  line L815 (13.0225, 4.201) -> (14.5225, 4.201)
  line L816 (14.5225, 4.201) -> (15.2725, 5.5)
  line L817 (18.0995, 7.25) -> (17.3495, 8.549)
  line L818 (17.3495, 8.549) -> (15.8495, 8.549)
  line L819 (15.8495, 8.549) -> (15.0995, 7.25)
  line L820 (15.0995, 7.25) -> (15.8495, 5.951)
  line L821 (17.3495, 5.951) -> (18.0995, 7.25)
  line L822 (15.8495, 5.951) -> (17.3495, 5.951)
  line L823 (-13, 9) -> (-13.75, 10.299)
  line L824 (-13.75, 10.299) -> (-15.25, 10.299)
  line L825 (-15.25, 10.299) -> (-16, 9)
  line L826 (-16, 9) -> (-15.25, 7.701)
  line L827 (-15.25, 7.701) -> (-13.75, 7.701)
  line L828 (-13.75, 7.701) -> (-13, 9)
  line L829 (-10.173, 10.75) -> (-10.923, 12.049)
  line L830 (-10.923, 12.049) -> (-12.423, 12.049)
  line L831 (-12.423, 12.049) -> (-13.173, 10.75)
  line L832 (-13.173, 10.75) -> (-12.423, 9.451)
  line L833 (-10.923, 9.451) -> (-10.173, 10.75)
  line L834 (-12.423, 9.451) -> (-10.923, 9.451)
  line L835 (-7.3455, 9) -> (-8.0955, 10.299)
  line L836 (-8.0955, 10.299) -> (-9.5955, 10.299)
  line L837 (-9.5955, 10.299) -> (-10.3455, 9)
  line L838 (-10.3455, 9) -> (-9.5955, 7.701)
  line L839 (-9.5955, 7.701) -> (-8.0955, 7.701)
  line L840 (-8.0955, 7.701) -> (-7.3455, 9)
  line L841 (-4.5185, 10.75) -> (-5.2685, 12.049)
  line L842 (-5.2685, 12.049) -> (-6.7685, 12.049)
  line L843 (-6.7685, 12.049) -> (-7.5185, 10.75)
  line L844 (-7.5185, 10.75) -> (-6.7685, 9.451)
  line L845 (-5.2685, 9.451) -> (-4.5185, 10.75)
  line L846 (-6.7685, 9.451) -> (-5.2685, 9.451)
  line L847 (-1.691, 9) -> (-2.441, 10.299)
  line L848 (-2.441, 10.299) -> (-3.941, 10.299)
  line L849 (-3.941, 10.299) -> (-4.691, 9)
  line L850 (-4.691, 9) -> (-3.941, 7.701)
  line L851 (-3.941, 7.701) -> (-2.441, 7.701)
  line L852 (-2.441, 7.701) -> (-1.691, 9)
  line L853 (1.136, 10.75) -> (0.386, 12.049)
  line L854 (0.386, 12.049) -> (-1.114, 12.049)
  line L855 (-1.114, 12.049) -> (-1.864, 10.75)
  line L856 (-1.864, 10.75) -> (-1.114, 9.451)
  line L857 (0.386, 9.451) -> (1.136, 10.75)
  line L858 (-1.114, 9.451) -> (0.386, 9.451)
  line L859 (3.9635, 9) -> (3.2135, 10.299)
  line L860 (3.2135, 10.299) -> (1.7135, 10.299)
  line L861 (1.7135, 10.299) -> (0.9635, 9)
  line L862 (0.9635, 9) -> (1.7135, 7.701)
  line L863 (1.7135, 7.701) -> (3.2135, 7.701)
  line L864 (3.2135, 7.701) -> (3.9635, 9)
  line L865 (6.7905, 10.75) -> (6.0405, 12.049)
  line L866 (6.0405, 12.049) -> (4.5405, 12.049)
  line L867 (4.5405, 12.049) -> (3.7905, 10.75)
  line L868 (3.7905, 10.75) -> (4.5405, 9.451)
  line L869 (6.0405, 9.451) -> (6.7905, 10.75)
  line L870 (4.5405, 9.451) -> (6.0405, 9.451)
  line L871 (9.618, 9) -> (8.868, 10.299)
  line L872 (8.868, 10.299) -> (7.368, 10.299)
  line L873 (7.368, 10.299) -> (6.618, 9)
  line L874 (6.618, 9) -> (7.368, 7.701)
  line L875 (7.368, 7.701) -> (8.868, 7.701)
  line L876 (8.868, 7.701) -> (9.618, 9)
  line L877 (12.445, 10.75) -> (11.695, 12.049)
  line L878 (11.695, 12.049) -> (10.195, 12.049)
  line L879 (10.195, 12.049) -> (9.445, 10.75)
  line L880 (9.445, 10.75) -> (10.195, 9.451)
  line L881 (11.695, 9.451) -> (12.445, 10.75)
  line L882 (10.195, 9.451) -> (11.695, 9.451)
  line L883 (15.2725, 9) -> (14.5225, 10.299)
  line L884 (14.5225, 10.299) -> (13.0225, 10.299)
  line L885 (13.0225, 10.299) -> (12.2725, 9)
  line L886 (12.2725, 9) -> (13.0225, 7.701)
  line L887 (13.0225, 7.701) -> (14.5225, 7.701)
  line L888 (14.5225, 7.701) -> (15.2725, 9)
  line L889 (18.0995, 10.75) -> (17.3495, 12.049)
  line L890 (17.3495, 12.049) -> (15.8495, 12.049)
  line L891 (15.8495, 12.049) -> (15.0995, 10.75)
  line L892 (15.0995, 10.75) -> (15.8495, 9.451)
  line L893 (17.3495, 9.451) -> (18.0995, 10.75)
  line L894 (15.8495, 9.451) -> (17.3495, 9.451)
  line L895 (-13, 12.5) -> (-13.75, 13.799)
  line L896 (-13.75, 13.799) -> (-15.25, 13.799)
  line L897 (-15.25, 13.799) -> (-16, 12.5)
  line L898 (-16, 12.5) -> (-15.25, 11.201)
  line L899 (-15.25, 11.201) -> (-13.75, 11.201)
  line L900 (-13.75, 11.201) -> (-13, 12.5)
  line L901 (-10.173, 14.25) -> (-10.923, 15.549)
  line L902 (-10.923, 15.549) -> (-12.423, 15.549)
  line L903 (-12.423, 15.549) -> (-13.173, 14.25)
  line L904 (-13.173, 14.25) -> (-12.423, 12.951)
  line L905 (-10.923, 12.951) -> (-10.173, 14.25)
  line L906 (-12.423, 12.951) -> (-10.923, 12.951)
  line L907 (-7.3455, 12.5) -> (-8.0955, 13.799)
  line L908 (-8.0955, 13.799) -> (-9.5955, 13.799)
  line L909 (-9.5955, 13.799) -> (-10.3455, 12.5)
  line L910 (-10.3455, 12.5) -> (-9.5955, 11.201)
  line L911 (-9.5955, 11.201) -> (-8.0955, 11.201)
  line L912 (-8.0955, 11.201) -> (-7.3455, 12.5)
  line L913 (-4.5185, 14.25) -> (-5.2685, 15.549)
  line L914 (-5.2685, 15.549) -> (-6.7685, 15.549)
  line L915 (-6.7685, 15.549) -> (-7.5185, 14.25)
  line L916 (-7.5185, 14.25) -> (-6.7685, 12.951)
  line L917 (-5.2685, 12.951) -> (-4.5185, 14.25)
  line L918 (-6.7685, 12.951) -> (-5.2685, 12.951)
  line L919 (-1.691, 12.5) -> (-2.441, 13.799)
  line L920 (-2.441, 13.799) -> (-3.941, 13.799)
  line L921 (-3.941, 13.799) -> (-4.691, 12.5)
  line L922 (-4.691, 12.5) -> (-3.941, 11.201)
  line L923 (-3.941, 11.201) -> (-2.441, 11.201)
  line L924 (-2.441, 11.201) -> (-1.691, 12.5)
  line L925 (1.136, 14.25) -> (0.386, 15.549)
  line L926 (0.386, 15.549) -> (-1.114, 15.549)
  line L927 (-1.114, 15.549) -> (-1.864, 14.25)
  line L928 (-1.864, 14.25) -> (-1.114, 12.951)
  line L929 (0.386, 12.951) -> (1.136, 14.25)
  line L930 (-1.114, 12.951) -> (0.386, 12.951)
  line L931 (3.9635, 12.5) -> (3.2135, 13.799)
  line L932 (3.2135, 13.799) -> (1.7135, 13.799)
  line L933 (1.7135, 13.799) -> (0.9635, 12.5)
  line L934 (0.9635, 12.5) -> (1.7135, 11.201)
  line L935 (1.7135, 11.201) -> (3.2135, 11.201)
  line L936 (3.2135, 11.201) -> (3.9635, 12.5)
  line L937 (6.7905, 14.25) -> (6.0405, 15.549)
  line L938 (6.0405, 15.549) -> (4.5405, 15.549)
  line L939 (4.5405, 15.549) -> (3.7905, 14.25)
  line L940 (3.7905, 14.25) -> (4.5405, 12.951)
  line L941 (6.0405, 12.951) -> (6.7905, 14.25)
  line L942 (4.5405, 12.951) -> (6.0405, 12.951)
  line L943 (9.618, 12.5) -> (8.868, 13.799)
  line L944 (8.868, 13.799) -> (7.368, 13.799)
  line L945 (7.368, 13.799) -> (6.618, 12.5)
  line L946 (6.618, 12.5) -> (7.368, 11.201)
  line L947 (7.368, 11.201) -> (8.868, 11.201)
  line L948 (8.868, 11.201) -> (9.618, 12.5)
  line L949 (12.445, 14.25) -> (11.695, 15.549)
  line L950 (11.695, 15.549) -> (10.195, 15.549)
  line L951 (10.195, 15.549) -> (9.445, 14.25)
  line L952 (9.445, 14.25) -> (10.195, 12.951)
  line L953 (11.695, 12.951) -> (12.445, 14.25)
  line L954 (10.195, 12.951) -> (11.695, 12.951)
  line L955 (15.2725, 12.5) -> (14.5225, 13.799)
  line L956 (14.5225, 13.799) -> (13.0225, 13.799)
  line L957 (13.0225, 13.799) -> (12.2725, 12.5)
  line L958 (12.2725, 12.5) -> (13.0225, 11.201)
  line L959 (13.0225, 11.201) -> (14.5225, 11.201)
  line L960 (14.5225, 11.201) -> (15.2725, 12.5)
  line L961 (18.0995, 14.25) -> (17.3495, 15.549)
  line L962 (17.3495, 15.549) -> (15.8495, 15.549)
  line L963 (15.8495, 15.549) -> (15.0995, 14.25)
  line L964 (15.0995, 14.25) -> (15.8495, 12.951)
  line L965 (17.3495, 12.951) -> (18.0995, 14.25)
  line L966 (15.8495, 12.951) -> (17.3495, 12.951)
  line L967 (-13, 16) -> (-13.75, 17.299)
  line L968 (-13.75, 17.299) -> (-15.25, 17.299)
  line L969 (-15.25, 17.299) -> (-16, 16)
  line L970 (-16, 16) -> (-15.25, 14.701)
  line L971 (-15.25, 14.701) -> (-13.75, 14.701)
  line L972 (-13.75, 14.701) -> (-13, 16)
  line L973 (-10.173, 17.75) -> (-10.923, 19.049)
  line L974 (-10.923, 19.049) -> (-12.423, 19.049)
  line L975 (-12.423, 19.049) -> (-13.173, 17.75)
  line L976 (-13.173, 17.75) -> (-12.423, 16.451)
  line L977 (-10.923, 16.451) -> (-10.173, 17.75)
  line L978 (-12.423, 16.451) -> (-10.923, 16.451)
  line L979 (-7.3455, 16) -> (-8.0955, 17.299)
  line L980 (-8.0955, 17.299) -> (-9.5955, 17.299)
  line L981 (-9.5955, 17.299) -> (-10.3455, 16)
  line L982 (-10.3455, 16) -> (-9.5955, 14.701)
  line L983 (-9.5955, 14.701) -> (-8.0955, 14.701)
  line L984 (-8.0955, 14.701) -> (-7.3455, 16)
  line L985 (-4.5185, 17.75) -> (-5.2685, 19.049)
  line L986 (-5.2685, 19.049) -> (-6.7685, 19.049)
  line L987 (-6.7685, 19.049) -> (-7.5185, 17.75)
  line L988 (-7.5185, 17.75) -> (-6.7685, 16.451)
  line L989 (-5.2685, 16.451) -> (-4.5185, 17.75)
  line L990 (-6.7685, 16.451) -> (-5.2685, 16.451)
  line L991 (-1.691, 16) -> (-2.441, 17.299)
  line L992 (-2.441, 17.299) -> (-3.941, 17.299)
  line L993 (-3.941, 17.299) -> (-4.691, 16)
  line L994 (-4.691, 16) -> (-3.941, 14.701)
  line L995 (-3.941, 14.701) -> (-2.441, 14.701)
  line L996 (-2.441, 14.701) -> (-1.691, 16)
  line L997 (1.136, 17.75) -> (0.386, 19.049)
  line L998 (0.386, 19.049) -> (-1.114, 19.049)
  line L999 (-1.114, 19.049) -> (-1.864, 17.75)
  line L1000 (-1.864, 17.75) -> (-1.114, 16.451)
  line L1001 (0.386, 16.451) -> (1.136, 17.75)
  line L1002 (-1.114, 16.451) -> (0.386, 16.451)
  line L1003 (3.9635, 16) -> (3.2135, 17.299)
  line L1004 (3.2135, 17.299) -> (1.7135, 17.299)
  line L1005 (1.7135, 17.299) -> (0.9635, 16)
  line L1006 (0.9635, 16) -> (1.7135, 14.701)
  line L1007 (1.7135, 14.701) -> (3.2135, 14.701)
  line L1008 (3.2135, 14.701) -> (3.9635, 16)
  line L1009 (6.7905, 17.75) -> (6.0405, 19.049)
  line L1010 (6.0405, 19.049) -> (4.5405, 19.049)
  line L1011 (4.5405, 19.049) -> (3.7905, 17.75)
  line L1012 (3.7905, 17.75) -> (4.5405, 16.451)
  line L1013 (6.0405, 16.451) -> (6.7905, 17.75)
  line L1014 (4.5405, 16.451) -> (6.0405, 16.451)
  line L1015 (9.618, 16) -> (8.868, 17.299)
  line L1016 (8.868, 17.299) -> (7.368, 17.299)
  line L1017 (7.368, 17.299) -> (6.618, 16)
  line L1018 (6.618, 16) -> (7.368, 14.701)
  line L1019 (7.368, 14.701) -> (8.868, 14.701)
  line L1020 (8.868, 14.701) -> (9.618, 16)
  line L1021 (12.445, 17.75) -> (11.695, 19.049)